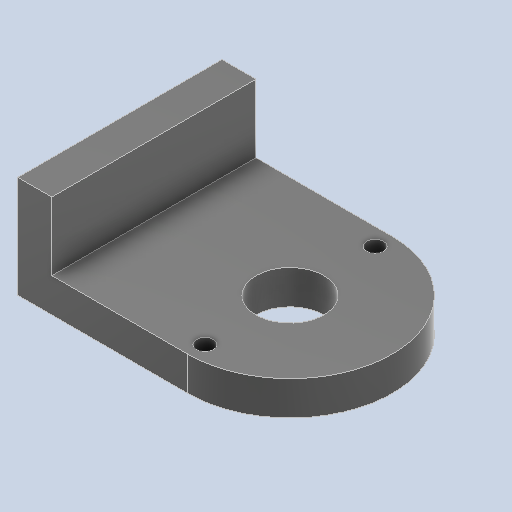
# Autodesk Inventor part: motor_mount
Saved by Autodesk Inventor 2022 (Build 260153000, 153)
## iProperties
Created: 2021-04-18
Part Number: motor_mount
Material: Plastic, Opaque Black
Document SubType Name: Modeling
Designer: kevin
Density: 0.952 g/cm^3
Appearance: Smooth - Black
Author: kevin
Autodesk Inventor part; units mm, degrees
ref_plane "YZ Plane" through (0, 0, 0) normal (1, 0, 0) x (0, 1, 0)
ref_plane "XZ Plane" through (0, 0, 0) normal (0, 1, 0) x (-1, 0, 0)
ref_plane "XY Plane" through (0, 0, 0) normal (0, 0, 1) x (1, 0, 0)
sketch "Sketch1" plane through (0, 0, 0) normal (0, 1, 0) x (-1, 0, 0)
  line L0 (-19.05, 19.05) -> (19.05, 19.05) construction
  line L1 (19.05, 19.05) -> (19.05, -19.05) construction
  line L2 (19.05, -19.05) -> (-19.05, -19.05) construction
  line L3 (-19.05, -19.05) -> (-19.05, 19.05) construction
  line L4 (-19.05, 19.05) -> (19.05, -19.05) construction
  line L5 (19.05, 19.05) -> (-19.05, -19.05) construction
  arc A0 (-19.05, 19.05) -> (-19.05, -19.05) centre (-19.05, 0) ccw
  circle A1 centre (-19.05, 0) radius 6.35
  circle A2 centre (-19.05, 15.875) radius 1.5875
  circle A3 centre (-19.05, -15.875) radius 1.5875
  line L6 (-17.4625, 15.875) -> (-17.4625, 19.05) construction
  line L7 (-17.4625, -15.875) -> (-17.4625, -19.05) construction
  line L8 (-19.05, 19.05) -> (0, 19.05)
  line L9 (0, -19.05) -> (-19.05, -19.05)
  line L10 (0, 19.05) -> (12.7, 19.05)
  line L11 (12.7, 19.05) -> (12.7, -19.05)
  line L12 (12.7, -19.05) -> (0, -19.05)
  line L13 (0, -19.05) -> (0, 19.05)
  line L14 (6.35, 19.05) -> (6.35, -19.05)
  line L15 (6.35, 9.525) -> (0, 9.525) construction
  point P0 (0, 0)
  dimension "d1" = 3.175
  dimension "d3" = 3.175
  dimension "d0" = 3.175
  dimension "d2" = 3.175
  dimension "d4" = 38.1
  dimension "d5" = 19.05
  dimension "d6" = 12.7
  dimension "d8" = 19.05
  dimension "d9" = 12.7
  dimension "d10" = 6.35
  constraints: 32 end point, 7 point on line, 6 midpoint, 6 perpendicular, 4 parallel, 2 centre point, 2 horizontal, 2 horizontal alignment, 2 point on circle, 2 vertical, 1 coincident, 4 other
  measures "d0" distance of L6.start L6.end
  measures "d2" distance of L7.start L7.end
  measures "d4" distance of L0.end L1.end
  measures "d5" radius of A0
  measures "d6" diameter of A1
  measures "d8" distance of L0.start L8.end
  measures "d9" distance of L11.end L12.end
  measures "d10" distance of L15.start L15.end
extrude "Extrusion1" add sketch "Sketch1" along normal blind 6.35
sketch "Sketch2" plane through (0, 6.35, 0) normal (0, 1, 0) x (1, 0, 0)
  line L0 (19.05, 19.05) -> (-12.7, 19.05) projected
  line L1 (-12.7, 19.05) -> (-6.35, 19.05)
  line L2 (-6.35, 19.05) -> (-6.35, -19.05)
  line L3 (-6.35, -19.05) -> (-12.7, -19.05)
  line L4 (-12.7, -19.05) -> (-12.7, 19.05)
  point P0 (0, 0)
  dimension "d16" = 6.35
  dimension "d17" = 38.1
  constraints: 8 end point, 2 parallel, 1 horizontal, 1 perpendicular
  measures "d16" distance of L2.end L3.end
  measures "d17" distance of L3.end L0.end
extrude "Extrusion2" add sketch "Sketch2" along normal blind 12.7
body "Solid1"
